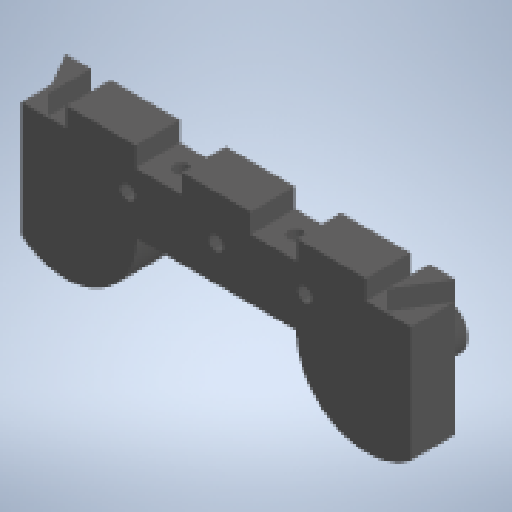
# Autodesk Inventor part: board_setter_upper
Saved by Autodesk Inventor 2024.1 (Build 281209000, 209)
## iProperties
Created: 2024-10-12
Part Number: board_setter_upper
Material: 一般
Document SubType Name: Modeling
Designer: hibik
Density: 1 g/cm^3
Appearance: 既定
Author: hibik
Autodesk Inventor part; units mm, degrees
ref_plane "YZ Plane" through (0, 0, 0) normal (1, 0, 0) x (0, 1, 0)
ref_plane "XZ Plane" through (0, 0, 0) normal (0, 1, 0) x (-1, 0, 0)
ref_plane "XY Plane" through (0, 0, 0) normal (0, 0, 1) x (1, 0, 0)
sketch "スケッチ1" plane through (0, 0, 0) normal (0, 0, 1) x (1, 0, 0)
  line L0 (-22, 30) -> (22, 30)
  line L1 (22, 30) -> (22, 0)
  line L2 (22, 0) -> (-22, 0)
  line L3 (-22, 0) -> (-22, 30)
  point P0 (0, 0)
  point P1 (0, 0)
  dimension "d0" = 30
  dimension "d1" = 44
  constraints: 8 end point, 2 parallel, 1 coincident, 1 horizontal, 1 midpoint, 1 perpendicular
  measures "d0" distance of L2.end L0.start
  measures "d1" distance of L0.start L0.end
extrude "押し出し1" add sketch "スケッチ1" along normal blind 5
sketch "スケッチ2" plane through (0, 0, 5) normal (0, 0, 1) x (1, 0, 0)
  arc A0 (-17, 13) -> (-13.5, 13.8063) centre (-17, 21) ccw
  arc A1 (-10.5, 16.3363) -> (-9, 21) centre (-17, 21) ccw
  line L0 (-7.5, 21) -> (-9, 21)
  line L1 (-1.5, 21) -> (-4.5, 21)
  arc A2 (9, 21) -> (10.5, 16.3363) centre (17, 21) ccw
  arc A3 (13.5, 13.8063) -> (17, 13) centre (17, 21) ccw
  circle A4 centre (-17, 21) radius 8
  circle A5 centre (17, 21) radius 8
  line L2 (-9, 21) -> (9, 21)
  line L3 (-22, 0) -> (22, 0)
  line L4 (22, 0) -> (22, 30)
  line L5 (22, 30) -> (-22, 30)
  line L6 (-22, 30) -> (-22, 0)
  point P0 (0, 0)
  point P1 (22, 14.755)
  point P2 (17, 13)
  point P3 (10.5, 16.3363)
  point P4 (-13.5, 13.8063)
  point P5 (-17, 13)
  point P6 (-22, 14.755)
extrude "押し出し2" cut sketch "スケッチ2" against normal through all contours A0 A4 A1 L0 L2 L1 A2 A5 A3 L4 L3 L6
sketch "スケッチ3" plane through (0, 0, 0) normal (0, 0, -1) x (-1, 0, 0)
  circle A0 centre (-17, 21) radius 3 projected
  circle A1 centre (17, 21) radius 3 projected
  circle A2 centre (-17, 21) radius 2.5
  circle A3 centre (17, 21) radius 2.5
  point P0 (0, 0)
  point P1 (-14.9, 18.325)
  dimension "d6" = 5
  dimension "d7" = 5
  constraints: 2 centre point, 2 coincident, 1 other
  measures "d6" diameter of A2
  measures "d7" diameter of A3
ref_plane "作業平面1" through (-20, -16, -4) normal (0, 0, 1) x (1, 0, 0)
extrude "押し出し3" add sketch "スケッチ3" along normal up to surface (4 mm away) contours A2 | A3
sketch "スケッチ6" plane through (0, 0, 5) normal (0, 0, 1) x (1, 0, 0)
  circle A0 centre (0, 25) radius 0.8 projected
  circle A1 centre (10, 25) radius 0.8 projected
  circle A2 centre (-10, 25) radius 0.8 projected
  point P0 (0, 0)
extrude "押し出し6" cut sketch "スケッチ6" against normal through all
